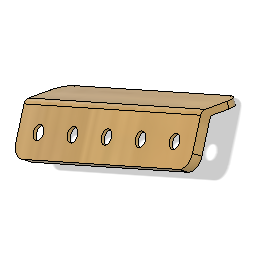
case_front (Autodesk Fusion 360 design; units mm, degrees)
Autodesk Fusion 360 part; units mm, degrees
sketch "Sketch1" plane through (0, 0, 0) normal (0, 1, 0) x (1, 0, 0)
  line L0 (-19.8209, 9.4872) -> (107.1791, 9.4872) construction
  line L1 (107.1791, 9.4872) -> (107.1791, -15.9128) construction
  line L2 (107.1791, -15.9128) -> (-19.8209, -15.9128) construction
  line L3 (-19.8209, -15.9128) -> (-19.8209, 9.4872) construction
  line L4 (43.6791, 9.4872) -> (43.6791, -15.9128) construction
  line L5 (107.1791, -3.2128) -> (-19.8209, -3.2128) construction
  line L6 (116.1791, -17.0528) -> (-28.8209, -17.0528)
  line L7 (-28.8209, -17.0528) -> (-28.8209, 12.9472)
  line L8 (-28.8209, 12.9472) -> (116.1791, 12.9472)
  line L9 (116.1791, 12.9472) -> (116.1791, -17.0528)
  circle A0 centre (43.6791, -3.2128) radius 4.2
  circle A1 centre (-12.2009, -3.2128) radius 4.2
  circle A2 centre (99.5591, -3.2128) radius 4.2
  circle A3 centre (15.7391, -3.2128) radius 4.2
  circle A4 centre (71.6191, -3.2128) radius 4.2
  point P0 (43.6791, -3.2128)
  dimension "d3" = 127
  dimension "d4" = 25.4
  dimension "d7" = 145
  dimension "d8" = 30
  dimension "d9" = 8.4
  dimension "d10" = 8.4
  dimension "d12" = 8.4
  dimension "d14" = 8.4
  dimension "d15" = 8.4
  dimension "d16" = 27.94
  dimension "d17" = 27.94
  dimension "d18" = 27.94
  dimension "d19" = 27.94
  dimension "d47" = 13.84
  constraint horizontal L0
  constraint vertical L1
  constraint horizontal L2
  constraint vertical L3
  constraint midpoint L0 L4.start
  constraint midpoint L2 L4.end
  constraint midpoint L1 L5.start
  constraint midpoint L3 L5.end
  constraint horizontal L6
  constraint perpendicular L6 L7
  constraint parallel L6 L8
  constraint parallel L7 L9
  constraint midpoint L4 P0
  constraint coincident P0 A0.centre
  constraint coincident L5 A1.centre
  constraint coincident L5 A2.centre
  constraint coincident L5 A3.centre
  constraint coincident L5 A4.centre
  measures "d3" distance of L0.start L0.end
  measures "d4" distance of L0.start L2.end
  measures "d7" distance of L7.end L8.end
  measures "d8" distance of L6.end L7.end
  measures "d9" diameter of A0
  measures "d10" diameter of A1
  measures "d12" diameter of A2
  measures "d14" diameter of A4
  measures "d15" diameter of A3
  measures "d16" distance of P0 A3.centre
  measures "d17" distance of P0 A4.centre
  measures "d18" distance of A2.centre A4.centre
  measures "d19" distance of A1.centre A3.centre
  measures "d47" distance of L5 L6
extrude "Extrude1" add sketch "Sketch1" along normal blind 4
sketch "Sketch2" plane through (116.1791, 0, 0) normal (1, 0, 0) x (0, 0, -1)
  line L0 (-17.0528, 0) -> (12.9472, 0)
  line L1 (12.9472, 0) -> (12.9472, 4)
  line L2 (12.9472, 4) -> (-17.0528, 4)
  line L3 (-17.0528, 4) -> (-17.0528, 0)
  line L4 (12.9472, 4) -> (25.266, -17.3367)
  line L5 (25.266, -17.3367) -> (21.8019, -19.3367)
  line L6 (21.8019, -19.3367) -> (8.3284, 4)
  dimension "d23" = 4
  dimension "d25" = 120
  constraint coincident L1.end L2.start
  constraint perpendicular L4 L5
  constraint coincident L2 L6.end
  constraint perpendicular L5 L6
  measures "d23" distance of L4.end L5.end
  measures "d25" angle of L2 L4
extrude "Extrude2" add sketch "Sketch2" against normal blind 145 contours L0 L1 L4 L5 L6
fillet "Fillet1" radius 8.4 2 edges at (-28.8209, 2, 17.0528) (116.1791, 2, 17.0528)
fillet "Fillet2" radius 8.4 2 edges at (-28.8209, -18.3367, -23.5339) (116.1791, -18.3367, -23.5339)
fillet "Fillet3" radius 4 1 edges at (43.6791, 4, -12.9472)
sketch "Sketch3" plane through (0, 0, 0) normal (0, -1, 0) x (1, 0, 0)
  arc A0 (116.1791, 8.6528) -> (107.7791, 17.0528) centre (107.7791, 8.6528) ccw
  line L0 (107.7791, 17.0528) -> (-20.4209, 17.0528)
  arc A1 (-20.4209, 17.0528) -> (-28.8209, 8.6528) centre (-20.4209, 8.6528) ccw
  line L1 (-28.8209, 8.6528) -> (-28.8209, -10.6378)
  line L2 (-28.8209, -10.6378) -> (116.1791, -10.6378)
  line L3 (116.1791, -10.6378) -> (116.1791, 8.6528)
  circle A2 centre (99.5591, 3.2128) radius 4.2
  circle A3 centre (43.6791, 3.2128) radius 4.2
  circle A4 centre (-12.2009, 3.2128) radius 4.2
  circle A5 centre (15.7391, 3.2128) radius 4.2
  circle A6 centre (71.6191, 3.2128) radius 4.2
  line L4 (-27.8209, -9.6378) -> (115.1791, -9.6378)
  line L5 (115.1791, -9.6378) -> (115.1791, 8.6528)
  arc A7 (115.1791, 8.6528) -> (107.7791, 16.0528) centre (107.7791, 8.6528) ccw
  line L6 (107.7791, 16.0528) -> (-20.4209, 16.0528)
  arc A8 (-20.4209, 16.0528) -> (-27.8209, 8.6528) centre (-20.4209, 8.6528) ccw
  line L7 (-27.8209, 8.6528) -> (-27.8209, -9.6378)
  constraint parallel L2 L4
  constraint parallel L3 L5
  constraint concentric A0 A7
  constraint parallel L0 L6
  constraint concentric A1 A8
  constraint parallel L1 L7
  constraint tangent A7 L6
  constraint tangent A8 L7
  constraint tangent L5 A7
  constraint tangent L6 A8
extrude "Extrude4" add sketch "Sketch3" along normal blind 2 contours A0 L0 A1 L1 L2 L3
draft "Draft1" angle -35 neutral plane through (116.1791, -19.3367, -21.8019) pull (0, -0.5, 0.866025) 1 faces at (19.5124, -0.6667, -10.6378)
fillet "Fillet5" radius 2 1 edges at (43.6791, -2, -11.7925)
extrude "Extrude5" cut 1 faces at (-23.952, 0, 0.3299) along direction (0, 1, 0) blind 2
extrude "Extrude3" [suppressed]
fillet "Fillet4" [suppressed]
equation "pcb_width = 127 mm" comment "width of pcb"
equation "pcb_length = 25.4 mm"
equation "d3 = pcb_width"
equation "d4 = pcb_length"
equation "dists_bw_pot_centres = 27.94 mm" comment "distance between potentiometer centres"
equation "m7_clearance = 8.4 mm" comment "clearance hole for m7, which is the pot clearance hole"
equation "d9 = m7_clearance"
equation "d10 = m7_clearance"
equation "d12 = m7_clearance"
equation "d14 = m7_clearance"
equation "d15 = m7_clearance"
equation "d16 = dists_bw_pot_centres"
equation "d17 = dists_bw_pot_centres"
equation "d18 = dists_bw_pot_centres"
equation "d19 = dists_bw_pot_centres"
equation "d20 = thickness"
equation "thickness = 4 mm"
equation "d23 = thickness"
equation "d25 = panel_angle"
equation "panel_angle = 120 deg"
equation "d30 = m7_clearance"
equation "d32 = m7_clearance"
equation "d34 = thickness"
named bodies: "main"
